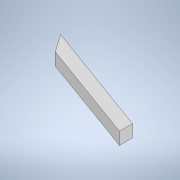
# Autodesk Inventor part: UpperInnerWD1
Saved by Autodesk Inventor 2020.1 (Build 241239000, 239)
## iProperties
Created: 2020-02-09
Part Number: UpperInnerWD1
Material: Generic
Document SubType Name: Modeling
Designer: super
Density: 1 g/cm^3
Appearance: Default
Author: super
Autodesk Inventor part; units mm, degrees
ref_plane "YZ Plane" through (0, 0, 0) normal (1, 0, 0) x (0, 1, 0)
ref_plane "XZ Plane" through (0, 0, 0) normal (0, 1, 0) x (-1, 0, 0)
ref_plane "XY Plane" through (0, 0, 0) normal (0, 0, 1) x (1, 0, 0)
sketch "Sketch1" plane through (0, 0, 0) normal (0, 1, 0) x (-1, 0, 0)
  line L0 (0, 0) -> (58.2609, -21.2052)
  line L1 (0, 0) -> (62, 0) construction
  line L2 (58.2609, -21.2052) -> (51.9109, -12.1365)
  line L3 (58.2609, -21.2052) -> (69.3318, -21.2052) construction
  line L4 (51.9109, -12.1365) -> (0, 6.7575)
  line L5 (0, 6.7575) -> (0, 0)
  dimension "d0" = 62
  dimension "d1" = 20
  dimension "d3" = 125
  constraints: 12 end point, 2 equal length, 2 horizontal, 1 point on line, 1 vertical
  measures "d0" distance of L0.start L0.end
  measures "d1" angle of L0 L1
  measures "d3" angle of L3 L2
extrude "Extrusion1" add sketch "Sketch1" along normal blind 6.35
body "Solid1"
